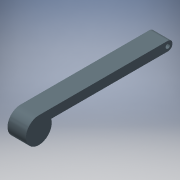
# Autodesk Inventor part: Arm
Saved by Autodesk Inventor 2016 (Build 200138000, 138)
## iProperties
Created: 2014-03-13
Part Number: Arm
Material: Lead
Document SubType Name: Modeling
Designer: John
Density: 1 g/cm^3
Appearance: Lead
Author: John
Autodesk Inventor part; units mm, degrees
ref_plane "YZ Plane" through (0, 0, 0) normal (1, 0, 0) x (0, 1, 0)
ref_plane "XZ Plane" through (0, 0, 0) normal (0, 1, 0) x (-1, 0, 0)
ref_plane "XY Plane" through (0, 0, 0) normal (0, 0, 1) x (1, 0, 0)
sketch "Sketch1" plane through (0, 0, 0) normal (1, 0, 0) x (0, 1, 0)
  line L0 (0, 0) -> (0, 44.45)
  arc A0 (0, 44.45) -> (-3.175, 40.1903) centre (-4.445, 44.45) ccw
  line L1 (-3.175, 40.1903) -> (-3.175, 0)
  line L2 (-3.175, 0) -> (0, 0)
  circle A1 centre (-1.5875, 0) radius 1.5875
  dimension "d0" = 3.175
  dimension "d1" = 44.45
  dimension "d2" = 4.445
  constraints: 6 end point, 2 point on circle, 1 centre point, 1 horizontal alignment, 1 midpoint, 1 parallel, 1 perpendicular, 1 tangent, 1 vertical, 2 other
  measures "d0" distance of L1.end L0.start
  measures "d1" distance of L0.start L0.end
  measures "d2" radius of A0
extrude "Extrusion1" add sketch "Sketch1" along normal blind 6.35
sketch "Sketch2" plane through (6.35, 0, 0) normal (1, 0, 0) x (0, 0, -1)
  arc A0 (0, -3.175) -> (0, 0) centre (0, -1.5875) ccw projected
hole "Hole1" at (6.35, -1.5875, 0) direction (-1, 0, 0) diameter 1.5875 end through all
body "Solid1"
